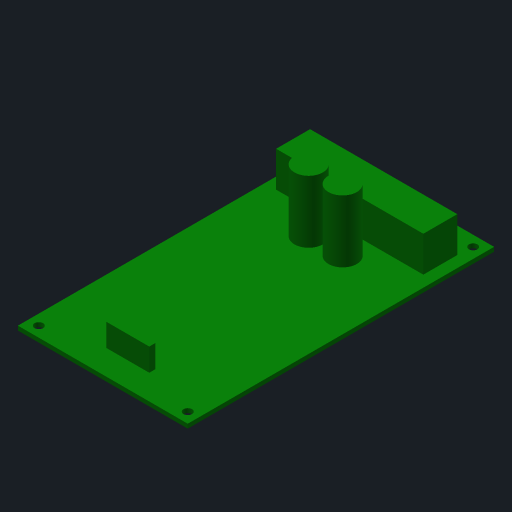
# Autodesk Inventor part: DRIVER
Saved by Autodesk Inventor 2024.3 (Build 283343000, 343)
## iProperties
Created: 2024-07-22
Part Number: DRIVER
Material: Steel, Mild, Welded
Document SubType Name: Modeling
Designer: Niler
Density: 7.85 g/cm^3
Appearance: Weld - Steel Mild
Author: Niler
Autodesk Inventor part; units mm, degrees
ref_plane "YZ Plane" through (0, 0, 0) normal (1, 0, 0) x (0, 1, 0)
ref_plane "XZ Plane" through (0, 0, 0) normal (0, 1, 0) x (-1, 0, 0)
ref_plane "XY Plane" through (0, 0, 0) normal (0, 0, 1) x (1, 0, 0)
sketch "Sketch1" plane through (0, 0, 0) normal (0, 1, 0) x (-1, 0, 0)
  line L0 (-30, 54.1) -> (30, 54.1)
  line L1 (30, 54.1) -> (30, -54.1)
  line L2 (30, -54.1) -> (-30, -54.1)
  line L3 (-30, -54.1) -> (-30, 54.1)
  line L4 (-30, 54.1) -> (30, -54.1) construction
  line L5 (30, 54.1) -> (-30, -54.1) construction
  circle A0 centre (26.3, 50.4) radius 1.5
  line L6 (0, 0) -> (11.9593, 0)
  line L7 (0, 0) -> (0, 9.8578)
  circle A1 centre (26.3, -50.4) radius 1.5
  circle A2 centre (-26.3, 50.4) radius 1.5
  circle A3 centre (-26.3, -50.4) radius 1.5
  dimension "d0" = 60
  dimension "d1" = 108.2
  dimension "d2" = 3.7
  dimension "d3" = 3.7
  dimension "d4" = 3
  constraints: 16 end point, 4 centre point, 3 symmetric about line, 2 horizontal, 2 midpoint, 2 parallel, 1 perpendicular, 1 vertical, 3 other
  measures "d0" distance of L1.end L2.end
  measures "d1" distance of L0.end L1.end
  measures "d2" distance from line of L1 A0.centre
  measures "d3" distance from line of L0 A0.centre
  measures "d4" diameter of A0
extrude "Extrusion1" add sketch "Sketch1" along normal blind 1.5
sketch "Sketch2" plane through (0, 1.5, 0) normal (0, 1, 0) x (1, 0, 0)
  line L0 (30, 54.1) -> (-30, 54.1) projected
  line L1 (-30, 54.1) -> (-30, -54.1) projected
  line L2 (-30, -54.1) -> (30, -54.1) projected
  line L3 (30, -54.1) -> (30, 54.1) projected
  circle A0 centre (26.3, 50.4) radius 1.5 projected
  circle A1 centre (26.3, -50.4) radius 1.5 projected
  circle A2 centre (-26.3, 50.4) radius 1.5 projected
  circle A3 centre (-26.3, -50.4) radius 1.5 projected
  line L4 (7.6, -45.3) -> (-7.6, -45.3)
  line L5 (-7.6, -45.3) -> (-7.6, -43.1)
  line L6 (-7.6, -43.1) -> (7.6, -43.1)
  line L7 (7.6, -43.1) -> (7.6, -45.3)
  line L8 (7.6, -45.3) -> (-7.6, -43.1) construction
  line L9 (-7.6, -45.3) -> (7.6, -43.1) construction
  point P0 (0, 0)
  point P1 (0, -44.2)
  point P2 (0, -54.1)
  dimension "d7" = 2.2
  dimension "d8" = 15.2
  dimension "d9" = 11
  constraints: 12 end point, 3 midpoint, 2 parallel, 1 horizontal, 1 perpendicular, 1 vertical alignment
  measures "d7" distance of L4.end L5.end
  measures "d8" distance of L5.end L6.end
  measures "d9" distance between parallel lines of L2 L6
extrude "Extrusion2" add sketch "Sketch2" along normal blind 8 contours L4 L5 L6 L7
sketch "Sketch3" plane through (0, 0, 0) normal (0, -1, 0) x (1, 0, 0)
  circle A0 centre (16.0331, -17.0211) radius 2.267
  circle A1 centre (-4.9851, -17.0211) radius 1.9033
  circle A2 centre (-1.7515, 17.0211) radius 2.2093
  circle A3 centre (16.0331, 36.153) radius 3.7001
  point P0 (0, 0)
  constraints: 4 centre point
extrude "Extrusion3" add sketch "Sketch3" along normal blind 2
sketch "Sketch4" plane through (0, 1.5, 0) normal (0, 1, 0) x (1, 0, 0)
  circle A0 centre (-6, 24.6) radius 5
  circle A1 centre (6, 24.6) radius 5
  line L0 (30, 54.1) -> (-30, 54.1) projected
  line L1 (-6, 24.6) -> (6, 24.6)
  point P0 (0, 0)
  point P1 (0, 24.6)
  point P2 (0, 54.1)
  dimension "d14" = 10
  dimension "d15" = 29.5
  dimension "d16" = 12
  constraints: 2 centre point, 2 end point, 2 midpoint, 1 equal radius, 1 horizontal, 1 horizontal alignment, 1 vertical alignment
  measures "d14" diameter of A0
  measures "d15" distance from line of L0 L1.start
  measures "d16" distance of L1.start L1.end
extrude "Extrusion4" add sketch "Sketch4" along normal blind 22
sketch "Sketch5" plane through (0, 1.5, 0) normal (0, 1, 0) x (1, 0, 0)
  circle A0 centre (6, 24.6) radius 5 projected
  circle A1 centre (-6, 24.6) radius 5 projected
  line L0 (7.6, -43.1) -> (7.6, -45.3) projected
  line L1 (7.6, -45.3) -> (-7.6, -45.3) projected
  line L2 (-7.6, -45.3) -> (-7.6, -43.1) projected
  line L3 (-7.6, -43.1) -> (7.6, -43.1) projected
  line L4 (30, 54.1) -> (-30, 54.1) projected
  line L5 (-30, 54.1) -> (-30, -54.1) projected
  line L6 (-30, -54.1) -> (30, -54.1) projected
  line L7 (30, -54.1) -> (30, 54.1) projected
  circle A2 centre (26.3, 50.4) radius 1.5 projected
  circle A3 centre (26.3, -50.4) radius 1.5 projected
  circle A4 centre (-26.3, 50.4) radius 1.5 projected
  circle A5 centre (-26.3, -50.4) radius 1.5 projected
  line L8 (26, 33.1) -> (-26, 33.1)
  line L9 (-26, 33.1) -> (-26, 45.1)
  line L10 (-26, 45.1) -> (26, 45.1)
  line L11 (26, 45.1) -> (26, 33.1)
  line L12 (26, 33.1) -> (-26, 45.1) construction
  line L13 (-26, 33.1) -> (26, 45.1) construction
  point P0 (0, 0)
  point P1 (0, 39.1)
  dimension "d19" = 52
  dimension "d20" = 12
  dimension "d21" = 9
  constraints: 12 end point, 2 midpoint, 2 parallel, 1 horizontal, 1 perpendicular, 1 vertical alignment
  measures "d19" distance of L9.end L10.end
  measures "d20" distance of L8.end L9.end
  measures "d21" distance between parallel lines of L4 L10
extrude "Extrusion5" add sketch "Sketch5" along normal blind 12.5 contours L8 L9 L10 L11
body "Solid1"
